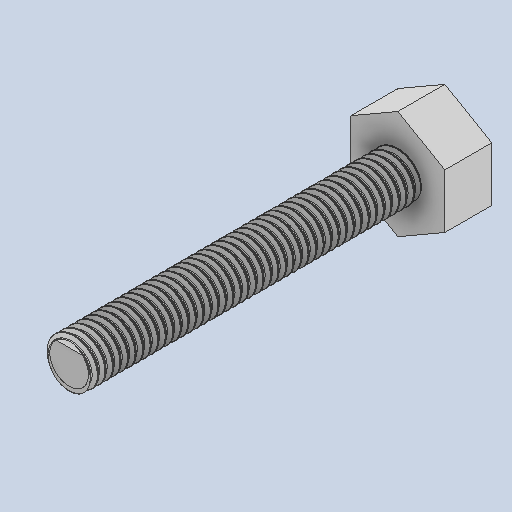
# Autodesk Inventor part: OutputFile
Saved by Autodesk Inventor 2023.1 (Build 271208000, 208)
## iProperties
Created: 2023-06-05
Part Number: OutputFile
Material: Generic
Document SubType Name: Modeling
Designer: Ronan
Density: 1 g/cm^3
Appearance: Default
Mass: 1.06712 g
Surface Area: 8.84096 cm^2
Volume: 1.06712 cm^3
Author: Ronan
Autodesk Inventor part; units mm, degrees
ref_plane "YZ Plane" through (0, 0, 0) normal (1, 0, 0) x (0, 1, 0)
ref_plane "XZ Plane" through (0, 0, 0) normal (0, 1, 0) x (-1, 0, 0)
ref_plane "XY Plane" through (0, 0, 0) normal (0, 0, 1) x (1, 0, 0)
sketch "Sketch1" plane through (0, 0, 0) normal (0, 0, 1) x (1, 0, 0)
  line L0 (5, 2.8868) -> (5, -2.8868)
  line L1 (5, 2.8868) -> (0, 5.7735)
  line L2 (-5, 2.8868) -> (0, 5.7735)
  line L3 (0, -5.7735) -> (5, -2.8868)
  line L4 (-5, 2.8868) -> (-5, -2.8868)
  line L5 (-5, -2.8868) -> (0, -5.7735)
  point P0 (0, 0)
  point P1 (0, 0)
  point P2 (0, 0)
  point P3 (0, 0)
  point P4 (0, 0)
  point P5 (0, 0)
  dimension "d0" = 120
  dimension "d1" = 120
  dimension "d2" = 120
  dimension "d3" = 120
  dimension "d4" = 120
  dimension "d5" = 120
  dimension "d6" = 10
  dimension "d7" = 5
  constraints: 12 end point, 3 coincident, 2 vertical
  measures "d0" angle of L3 L0
  measures "d1" angle of L5 L3
  measures "d2" angle of L5 L4
  measures "d3" angle of L4 L2
  measures "d4" angle of L2 L1
  measures "d5" angle of L1 L0
  measures "d6" distance between parallel lines of L0 L4
  measures "d7" distance from line of L4 point (0, 0)
extrude "Extrusion1" add sketch "Sketch1" along normal blind 5
sketch "Sketch2" plane through (0, 0, 5) normal (0, 0, 1) x (1, 0, 0)
  circle A0 centre (0, 0) radius 2.5
  dimension "d10" = 5
  constraints: 1 centre point, 1 coincident
  measures "d10" diameter of A0
extrude "Extrusion2" add sketch "Sketch2" along normal blind 35
thread "Thread1" size "M5x0.8" class "6g" standard "ANSI Metric M Profile" full length
sketch "Sketch3" plane through (0, 0, 40) normal (0, 0, 1) x (1, 0, 0)
  line L0 (0, 0) -> (0, 1.5)
  line L1 (0, 1.5) -> (2, 1.5)
  line L2 (2, 1.5) -> (-2, 1.5)
  circle A0 centre (0, 0) radius 2.5 projected
  circle A1 centre (0, 0) radius 2.5
  dimension "d15" = 1.5
  constraints: 6 end point, 1 coincident, 1 perpendicular, 1 point on line, 1 vertical, 5 other
  measures "d15" distance of L0.start L0.end
extrude "Extrusion3" cut sketch "Sketch3" against normal blind 19 contours L2 A0 L1 picked at (-1.2006, 1.6398)
sketch "Sketch5" plane through (0, 0, 40) normal (-1, 0, 0) x (0, 1, 0)
  line L0 (2.5, 0) -> (2.5, 35)
  line L1 (2.5, 35) -> (2.067, 35)
  line L2 (2.067, 35) -> (2.067, 0)
  line L3 (2.067, 0) -> (2.5, 0)
  line L4 (0, -9.02) -> (0, 48.17) projected
  constraints: 8 end point
revolve "Revolution1" cut sketch "Sketch5" angle 360 about axis through (0, 0, 40) along (0, 0, -1)
sketch "Sketch6" plane through (0, 0, 40) normal (-1, 0, 0) x (0, 1, 0)
  line L0 (2.5, 0) -> (2.5, 35)
  line L1 (2.5, 35) -> (2.067, 35)
  line L2 (2.067, 35) -> (2.067, 0)
  line L3 (2.067, 0) -> (2.5, 0)
  line L4 (0, -9.02) -> (0, 48.17) projected
  constraints: 8 end point
revolve "Revolution2" add sketch "Sketch6" angle 360 about axis through (0, 0, 40) along (0, 0, -1) separate body
sketch "Sketch4" plane through (0, 0, 40) normal (1, 0, 0) x (0, 0, -1)
  line L0 (-0.4, -1.8938) -> (-0.5289, -2.117) construction
  line L1 (-0.4, -1.8938) -> (-0.2711, -2.117) construction
  line L2 (-0.4, -1.8938) -> (-0.4, -2.067) construction
  line L3 (-0.5, -2.067) -> (-0.4423, -2.067) construction
  line L4 (0, -2.5866) -> (0.05, -2.5) construction
  line L5 (-0.8, -2.5866) -> (-0.85, -2.5) construction
  line L6 (-0.85, -2.5) -> (-0.8, -2.5) construction
  line L7 (-0.75, -2.5) -> (-0.8, -2.5866) construction
  arc A0 (-0.4423, -2.067) -> (-0.5289, -2.117) centre (-0.4423, -2.167) ccw
  arc A1 (-0.2711, -2.117) -> (-0.3577, -2.067) centre (-0.3577, -2.167) ccw
  line L8 (0, -2.5866) -> (0, -2.5) construction
  line L9 (-0.8, -2.5866) -> (-0.8, -2.5) construction
  arc A2 (-0.0644, -2.475) -> (-0.0211, -2.5) centre (-0.0211, -2.45) ccw
  line L10 (-0.2711, -2.117) -> (-0.0644, -2.475)
  line L11 (-0.4423, -2.067) -> (-0.3577, -2.067)
  line L12 (-0.5289, -2.117) -> (-0.7356, -2.475)
  line L13 (-0.0211, -2.5) -> (0, -2.5) construction
  line L14 (0, -2.5) -> (0.05, -2.5) construction
  arc A3 (-0.7789, -2.5) -> (-0.7356, -2.475) centre (-0.7789, -2.45) ccw
  line L15 (-0.7356, -2.475) -> (-0.75, -2.5) construction
  line L16 (-0.8, -2.5) -> (-0.7789, -2.5) construction
  line L17 (-0.7789, -2.5) -> (-0.0211, -2.5)
  line L18 (0, 0) -> (0.4413, 0)
  line L19 (0, 0) -> (0, 0.419)
  line L20 (0, -2.5866) -> (-0.0644, -2.475) construction
  dimension "d18" = 0.1732
  dimension "d19" = 0.1
  dimension "d20" = 0.05
  dimension "d21" = 0.0866
  dimension "d22" = 0.8
  dimension "Sketch4_MajorRadius" = 2.5
  dimension "d24" = 60
  dimension "Sketch4_ThreadOffset" = 0
  dimension "Sketch4_MinorRadius" = 2.067
  constraints: 42 end point, 17 tangent, 8 point on circle, 6 parallel, 5 collinear, 4 centre point, 3 point on line, 3 vertical, 2 equal radius, 2 horizontal, 2 perpendicular, 1 equal length, 1 midpoint, 4 other
  measures "d18" distance from line of L0.start L3
  measures "d19" radius of A0
  measures "d20" radius of A2
  measures "d21" distance from line of L14 L4.start
  measures "d22" distance between parallel lines of L8 L9
  measures "Sketch4_MajorRadius" distance between parallel lines of L14 L18
  measures "d24" angle of L10 L12
  measures "Sketch4_ThreadOffset" distance between parallel lines of L19 L8
  measures "Sketch4_MinorRadius" distance between parallel lines of L18 L11
coil "Coil1" sketch "Sketch4" operation cut axis through (0, 0, 40) along (0, 0, -1) pitch 0.8008 turns 45.704296 hand right bodies 2
equation "\"d18\" = 0.216506 * Sketch4_Pitch"
equation "\"d19\" = d27"
equation "\"d20\" = 0.0625 * Sketch4_Pitch"
equation "\"d21\" = 0.108253 * Sketch4_Pitch"
equation "\"d22\" = Sketch4_Pitch"
equation "\"d24\" = d29"
equation "\"d27\" = 0.125 * Sketch4_Pitch"
equation "\"Sketch4_Pitch\" = 0.8"
equation "\"d29\" = 60deg"
body "Solid1"
body "Solid2"
